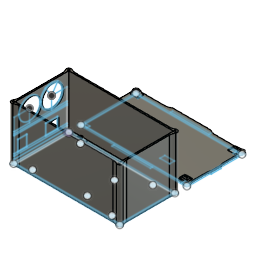
(CAD) Case Shield DMX Arduino Mega (Autodesk Fusion 360 design; units mm, degrees)
Autodesk Fusion 360 part; units mm, degrees
ref_plane "Plan de construction1" through (0, 0, 0) normal (0, 1, 0) x (0, 0, 1)
sketch "Esquisse1" plane through (0, 0, 0) normal (0, 1, 0) x (1, 0, 0)
  line L0 (0, 0) -> (108, 0)
  line L1 (108, 0) -> (108, -55)
  line L2 (108, -55) -> (0, -55)
  line L3 (0, -55) -> (0, 0)
  circle A0 centre (14, -51.75) radius 1
  circle A1 centre (15.25, -3.25) radius 1
  circle A2 centre (90.5, -3) radius 1
  circle A3 centre (96.75, -51.75) radius 1
  circle A4 centre (66, -18.5) radius 1
  circle A5 centre (66, -46.75) radius 1
  line L4 (-0.5, 0.5) -> (108.5, 0.5)
  line L5 (108.5, 0.5) -> (108.5, -55.5)
  line L6 (108.5, -55.5) -> (-0.5, -55.5)
  line L7 (-0.5, -55.5) -> (-0.5, 0.5)
  line L8 (-2, 2) -> (110, 2)
  line L9 (110, 2) -> (110, -57)
  line L10 (110, -57) -> (-2, -57)
  line L11 (-2, -57) -> (-2, 2)
  circle A6 centre (109.25, 1.25) radius 1
  circle A7 centre (109.25, 1.25) radius 2.5
  circle A8 centre (-1.25, 1.25) radius 1
  circle A9 centre (-1.25, 1.25) radius 2.5
  circle A10 centre (-1.25, -56.25) radius 1
  circle A11 centre (-1.25, -56.25) radius 2.5
  circle A12 centre (109.25, -56.25) radius 1
  circle A13 centre (109.25, -56.25) radius 2.5
  circle A14 centre (15.25, -3.25) radius 2
  circle A15 centre (66, -18.5) radius 2
  circle A16 centre (90.5, -3) radius 2
  circle A17 centre (96.75, -51.75) radius 2
  circle A18 centre (66, -46.75) radius 2
  circle A19 centre (14, -51.75) radius 2
  circle A20 centre (15.25, -3.25) radius 1.4
  circle A21 centre (90.5, -3) radius 1.4
  circle A22 centre (66, -18.5) radius 1.4
  circle A23 centre (96.75, -51.75) radius 1.4
  circle A24 centre (66, -46.75) radius 1.4
  circle A25 centre (14, -51.75) radius 1.4
  dimension "d23" = 2.8
  dimension "d24" = 2.8
  dimension "d25" = 2.8
  dimension "d26" = 2.8
  dimension "d27" = 2.8
  dimension "d28" = 2.8
  constraint horizontal L0
  constraint vertical L1
  constraint horizontal L2
  constraint vertical L3
  constraint coincident L0.start L3.end
  constraint horizontal L4
  constraint vertical L5
  constraint horizontal L6
  constraint vertical L7
  constraint horizontal L8
  constraint vertical L9
  constraint horizontal L10
  constraint vertical L11
  constraint concentric A6 A7
  constraint concentric A8 A9
  constraint concentric A10 A11
  constraint concentric A12 A13
  constraint concentric A1 A14
  constraint concentric A4 A15
  constraint concentric A2 A16
  constraint concentric A3 A17
  constraint concentric A5 A18
  constraint concentric A0 A19
  constraint concentric A1 A20
  constraint concentric A16 A21
  constraint concentric A4 A22
  constraint concentric A17 A23
  constraint concentric A18 A24
  constraint concentric A0 A25
  measures "d23" diameter of A20
  measures "d24" diameter of A21
  measures "d25" diameter of A22
  measures "d26" diameter of A23
  measures "d27" diameter of A24
  measures "d28" diameter of A25
extrude "Extrusion1" add sketch "Esquisse1" along normal blind 3 contours L0 L3 L4 L7 A9 | L0 L3 A9 | L0 L4 A7 A9 | L0 L1 L2 L3 A7 A9 A11 A13 | L3 L7 A9 A11 | L0 L1 L4 L5 A7 | L0 L1 A7 | L4 L8 A7 A9 | L4 L7 L8 L11 A8 A9 | L2 L3 A11 | L2 L3 L6 L7 A11 | L7 L11 A9 A11 | L4 L5 L8 L9 A6 A7 | L1 L5 A7 A13 | L2 L6 A11 A13 | L6 L7 L10 L11 A10 A11 | L8 L11 A8 A9 | L8 L9 A6 A7 | L1 L2 L5 L6 A13 | L1 L2 A13 | L5 L9 A7 A13 | L6 L10 A11 A13 | L10 L11 A10 A11 | L11 A8 | L8 L11 A8 | L8 A6 | L8 L9 A6 | L5 L6 L9 L10 A12 A13 | L8 A8 | L10 L11 A10 | L11 A10 | L8 L11 A8 | L8 L9 A6 | L9 A6 | L9 L10 A12 A13 | L10 L11 A10 | L10 A10 | L9 A12 | L9 L10 A12 | L10 A12 | L9 L10 A12 | A0 | A1 | A2 | A3 | A4 | A5 | A14 | A15 | A16 | A17 | A18 | A19 | A20 | A21 | A22 | A23 | A24 | A25 makes body 1
extrude "Extrusion2" add sketch "Esquisse1" along normal blind 56 contours L4 L8 A7 A9 | L4 L7 L8 L11 A8 A9 | L7 L11 A9 A11 | L4 L5 L8 L9 A6 A7 | L6 L7 L10 L11 A10 A11 | L8 L11 A8 A9 | L8 L9 A6 A7 | L5 L9 A7 A13 | L6 L10 A11 A13 | L10 L11 A10 A11 | L5 L6 L9 L10 A12 A13 | L8 L11 A8 | L8 L9 A6 | L9 L10 A12 A13 | L10 L11 A10 | L9 L10 A12 picked at (-1.9713, 1.9713) picked at (109.9713, 1.9713) picked at (-1.9713, -56.9713) picked at (109.9713, -56.9713) bodies 1
extrude "Extrusion3" add sketch "Esquisse1" along normal blind 40 contours L11 A8 | L8 L11 A8 | L8 A6 | L8 L9 A6 | L8 A8 | L10 L11 A10 | L11 A10 | L9 A6 | L10 A10 | L9 A12 | L9 L10 A12 | L10 A12 picked at (-1.4965, 1.4664) picked at (109.2357, 1.417) picked at (-1.3833, -56.1083) picked at (109.4133, -56.1968) bodies 1
extrude "Extrusion4" add sketch "Esquisse1" along normal blind 6 contours A14 | A15 | A16 | A17 | A18 | A19 | A20 | A21 | A22 | A23 | A24 | A25 bodies 1
ref_plane "Plan de construction2" through (-2, 28, 27.5) normal (-1, 0, 0) x (0, 0, 1)
sketch "Esquisse2" plane through (-2, 0, 0) normal (-1, 0, 0) x (0, 0, 1)
  line L0 (0, 0) -> (55, 0)
  line L1 (55, 0) -> (55, 3)
  line L2 (55, 3) -> (0, 3)
  line L3 (0, 3) -> (0, 0)
  line L4 (0, 3) -> (55, 3)
  line L5 (55, 3) -> (55, 6)
  line L6 (55, 6) -> (0, 6)
  line L7 (0, 6) -> (0, 3)
  line L8 (0, 6) -> (55, 6)
  line L9 (55, 6) -> (55, 8)
  line L10 (55, 8) -> (0, 8)
  line L11 (0, 8) -> (0, 6)
  line L12 (10, 8) -> (22, 8)
  line L13 (22, 8) -> (22, 19)
  line L14 (22, 19) -> (10, 19)
  line L15 (10, 19) -> (10, 8)
  line L16 (51, 8) -> (42, 8)
  line L17 (42, 8) -> (42, 19)
  line L18 (42, 19) -> (51, 19)
  line L19 (51, 19) -> (51, 8)
  line L20 (9.8, 19.2) -> (22.2, 19.2)
  line L21 (22.2, 19.2) -> (22.2, 7.8)
  line L22 (22.2, 7.8) -> (9.8, 7.8)
  line L23 (9.8, 7.8) -> (9.8, 19.2)
  line L24 (41.8, 7.8) -> (51.2, 7.8)
  line L25 (51.2, 7.8) -> (51.2, 19.2)
  line L26 (51.2, 19.2) -> (41.8, 19.2)
  line L27 (41.8, 19.2) -> (41.8, 7.8)
  line L28 (0, 8) -> (55, 8)
  line L29 (55, 8) -> (55, 24.5)
  line L30 (55, 24.5) -> (0, 24.5)
  line L31 (0, 24.5) -> (0, 8)
  line L32 (0, 24.5) -> (55, 24.5)
  line L33 (55, 24.5) -> (55, 26)
  line L34 (55, 26) -> (0, 26)
  line L35 (0, 26) -> (0, 24.5)
  line L36 (0, 26) -> (55, 26)
  line L37 (55, 26) -> (55, 28)
  line L38 (55, 28) -> (0, 28)
  line L39 (0, 28) -> (0, 26)
  line L40 (0, 28) -> (16, 28)
  line L41 (16, 28) -> (16, 41)
  line L42 (16, 41) -> (0, 41)
  line L43 (0, 41) -> (0, 28)
  line L44 (55, 28) -> (39, 28)
  line L45 (39, 28) -> (39, 41)
  line L46 (39, 41) -> (55, 41)
  line L47 (55, 41) -> (55, 28)
  circle A0 centre (16, 41) radius 11
  circle A1 centre (39, 41) radius 11
  circle A2 centre (16, 41) radius 11.1
  circle A3 centre (39, 41) radius 11.1
  circle A4 centre (16, 41) radius 12
  line L48 (9.4651, 51.0645) -> (22.5349, 51.0645)
  line L49 (16, 41) -> (22.5349, 51.0645)
  line L50 (16, 41) -> (9.4651, 51.0645)
  constraint horizontal L0
  constraint vertical L1
  constraint horizontal L2
  constraint vertical L3
  constraint coincident L0.start L3.end
  constraint horizontal L4
  constraint vertical L5
  constraint horizontal L6
  constraint vertical L7
  constraint horizontal L8
  constraint vertical L9
  constraint horizontal L10
  constraint vertical L11
  constraint horizontal L12
  constraint vertical L13
  constraint horizontal L14
  constraint vertical L15
  constraint coincident L10 L12.start
  constraint horizontal L16
  constraint vertical L17
  constraint horizontal L18
  constraint vertical L19
  constraint coincident L10 L16.start
  constraint horizontal L20
  constraint vertical L21
  constraint horizontal L22
  constraint vertical L23
  constraint horizontal L24
  constraint vertical L25
  constraint horizontal L26
  constraint vertical L27
  constraint horizontal L28
  constraint vertical L29
  constraint horizontal L30
  constraint vertical L31
  constraint horizontal L32
  constraint vertical L33
  constraint horizontal L34
  constraint vertical L35
  constraint horizontal L36
  constraint vertical L37
  constraint horizontal L38
  constraint vertical L39
  constraint horizontal L40
  constraint vertical L41
  constraint horizontal L42
  constraint vertical L43
  constraint horizontal L44
  constraint vertical L45
  constraint horizontal L46
  constraint vertical L47
  constraint coincident L41.end L42.start
  constraint coincident L45.end L46.start
  constraint concentric A0 A2
  constraint concentric A1 A3
  constraint concentric A2 A4
  constraint coincident A4 L48.start
  constraint coincident A4 L48.end
  constraint horizontal L48
extrude "Extrusion5" cut sketch "Esquisse2" against normal blind 2 contours L10 L13 L14 L15 L20 L21 L23 L28 | L10 L12 L21 L22 L23 L28 | L10 L12 L13 L14 L15 L28 bodies 1
extrude "Extrusion6" cut sketch "Esquisse2" against normal blind 2 contours L10 L16 L24 L25 L27 L28 | L10 L17 L18 L19 L25 L26 L27 L28 | L10 L16 L17 L18 L19 L28 bodies 1
extrude "Extrusion7" cut sketch "Esquisse2" against normal blind 2 contours L41 L42 A0 A2 | L41 A0 A2 L49 | L42 A0 A2 L50 | A2 A4 L48 | A2 L48 L50 | L41 L42 A0 | L41 A0 L49 | L42 A0 L50 | A0 A2 L48 L50 | A2 L48 L49 | A0 A2 L48 | A0 L48 L49 L50 | A0 A2 L48 L49 | A0 L48 bodies 1
extrude "Extrusion8" cut sketch "Esquisse2" against normal blind 2 contours L45 A1 A3 A4 | L45 L46 A1 A3 | L46 A1 A3 A4 | A3 A4 | L45 L46 A1 | L45 L46 A1 bodies 1
fillet "Congé1" radius 10 8 edges at (-2, 28, 1.1348) (-2, 28, 53.8652) (1.1348, 28, -2) (106.8651, 28, -2) (110, 28, 1.1348) (110, 28, 53.8652) (1.1348, 28, 57) (106.8652, 28, 57) on bodies 1
fillet "Congé2" radius 3 6 edges at (13.3853, 3, 2.5268) (64.1353, 3, 17.7768) (88.6353, 3, 2.2768) (94.8853, 3, 51.0268) (64.1353, 3, 46.0268) (12.1353, 3, 51.0268) on bodies 1
extrude "Extrusion9" add sketch "Esquisse1" along normal blind 7.5 contours A20 | A21 | A22 | A23 | A24 | A25 bodies 1
extrude "Extrusion10" cut 2 faces at (15.1064, 7.5, 52.36) (16.5115, 7.5, 3.3196) along direction (0, -1, 0) blind 1.5 on bodies 1 bodies 1
sketch "Esquisse3" plane through (0, 0, 0) normal (0, 1, 0) x (1, 0, 0)
  circle A0 centre (-1.25, 13.75) radius 2.5
  circle A1 centre (-1.25, 13.75) radius 1
  line L0 (110, 13) -> (-2, 13)
  line L1 (-2, 13) -> (-2, 72)
  line L2 (108.6, 14.4) -> (-0.6, 14.4)
  line L3 (-0.6, 14.4) -> (-0.6, 70.6)
  line L4 (108, 15) -> (0, 15)
  line L5 (0, 15) -> (0, 70)
  circle A2 centre (-1.25, 71.25) radius 2.5
  circle A3 centre (-1.25, 71.25) radius 1
  line L6 (-0.6, 70.6) -> (108.6, 70.6)
  line L7 (-2, 72) -> (110, 72)
  line L8 (0, 70) -> (108, 70)
  circle A4 centre (109.25, 71.25) radius 2.5
  line L9 (108, 70) -> (108, 15)
  line L10 (108.6, 70.6) -> (108.6, 14.4)
  line L11 (110, 72) -> (110, 13)
  circle A5 centre (109.25, 71.25) radius 1
  circle A6 centre (109.25, 13.75) radius 2.5
  circle A7 centre (109.25, 13.75) radius 1
  line L12 (74, 72) -> (34, 72)
  line L13 (34, 72) -> (34, 74)
  line L14 (34, 74) -> (74, 74)
  line L15 (74, 74) -> (74, 72)
  line L16 (74, 13) -> (34, 13)
  line L17 (34, 13) -> (34, 11)
  line L18 (34, 11) -> (74, 11)
  line L19 (74, 11) -> (74, 13)
  line L20 (110, 47.5) -> (111, 47.5)
  line L21 (111, 47.5) -> (111, 37.5)
  line L22 (111, 37.5) -> (110, 37.5)
  line L23 (110, 37.5) -> (110, 47.5)
  line L24 (108.6, 70.6) -> (103.6, 70.6)
  line L25 (103.6, 70.6) -> (103.6, 67.6)
  line L26 (103.6, 67.6) -> (108.6, 67.6)
  line L27 (108.6, 67.6) -> (108.6, 70.6)
  line L28 (108.6, 14.4) -> (103.5, 14.4)
  line L29 (103.5, 14.4) -> (103.5, 17.5)
  line L30 (103.5, 17.5) -> (108.6, 17.5)
  line L31 (108.6, 17.5) -> (108.6, 14.4)
  line L32 (-0.6, 14.4) -> (4.4, 14.4)
  line L33 (4.4, 14.4) -> (4.4, 17.4)
  line L34 (4.4, 17.4) -> (-0.6, 17.4)
  line L35 (-0.6, 17.4) -> (-0.6, 14.4)
  line L36 (-0.6, 70.6) -> (4.5, 70.6)
  line L37 (4.5, 70.6) -> (4.5, 67.5)
  line L38 (4.5, 67.5) -> (-0.6, 67.5)
  line L39 (-0.6, 67.5) -> (-0.6, 70.6)
  line L40 (70, 25) -> (80, 25)
  line L41 (80, 25) -> (80, 30)
  line L42 (80, 30) -> (70, 30)
  line L43 (70, 30) -> (70, 25)
  constraint horizontal L8
  constraint vertical L9
  constraint horizontal L4
  constraint vertical L5
  constraint horizontal L6
  constraint vertical L10
  constraint horizontal L2
  constraint vertical L3
  constraint horizontal L7
  constraint vertical L11
  constraint horizontal L0
  constraint vertical L1
  constraint concentric A4 A5
  constraint concentric A2 A3
  constraint concentric A0 A1
  constraint concentric A6 A7
  constraint horizontal L12
  constraint vertical L13
  constraint horizontal L14
  constraint vertical L15
  constraint coincident L7 L12.start
  constraint horizontal L16
  constraint vertical L17
  constraint horizontal L18
  constraint vertical L19
  constraint coincident L0 L16.start
  constraint horizontal L20
  constraint vertical L21
  constraint horizontal L22
  constraint vertical L23
  constraint coincident L11 L20.start
  constraint horizontal L24
  constraint vertical L25
  constraint horizontal L26
  constraint vertical L27
  constraint horizontal L28
  constraint vertical L29
  constraint horizontal L30
  constraint vertical L31
  constraint horizontal L32
  constraint vertical L33
  constraint horizontal L34
  constraint vertical L35
  constraint horizontal L36
  constraint vertical L37
  constraint horizontal L38
  constraint vertical L39
  constraint horizontal L40
  constraint vertical L41
  constraint horizontal L42
  constraint vertical L43
extrude "Extrusion12" add sketch "Esquisse3" along normal blind 3 separate body contours A0 A1 L0 L2 L32 | A0 L0 L2 A6 L16 L28 L32 | A0 A1 L2 L3 L4 L5 L32 L35 | A0 L2 L4 L32 L33 | A0 A1 L0 L1 | A0 L4 L5 | A0 L4 L5 L33 L34 | L2 L4 L29 L33 | A1 L2 L3 L32 L35 | A1 L0 L1 L2 L3 L32 L35 | A0 L1 L3 A2 L35 L39 | A0 A1 L1 L3 L35 | L0 L16 L17 L18 L19 | A1 L0 | A0 L3 L5 L34 L35 | L4 L5 L8 L9 L25 L26 L29 L30 L33 L34 L37 L38 | L2 L4 A6 L28 L29 | A1 L1 | L1 A2 A3 L7 | L1 L3 A2 A3 L39 | A1 L0 L1 | L3 L5 L34 L38 | L4 L9 A6 L29 L30 | L2 L4 L9 L10 A6 A7 L28 L31 | L0 L2 A6 A7 L28 | L1 A3 | L1 L3 A3 L6 L7 L36 L39 | A2 L6 L7 A4 L12 L24 L36 | A2 A3 L6 L7 L36 | L3 L5 A2 L38 L39 | L3 L5 A2 A3 L6 L8 L36 L39 | L0 L11 A6 A7 | L5 A2 L8 L37 L38 | L4 L9 A6 | L2 L10 A7 L28 L31 | L0 L2 L10 L11 A7 L28 L31 | L1 A3 L7 | L3 A3 L6 L36 L39 | A3 L7 | L7 L12 L13 L14 L15 | L5 A2 L8 | L0 A7 | L9 L10 A6 L30 L31 | L9 L10 L26 L30 | L10 L11 A6 A7 L31 | A2 L6 L8 L36 L37 | L0 L11 A7 | A4 L10 L11 A6 L23 L27 L31 | L6 L8 L25 L37 | L8 A4 L9 L25 L26 | A4 L9 L10 L26 L27 | L11 A7 | L7 A4 L11 A5 | L6 L7 A4 A5 L24 | L11 L20 L21 L22 L23 | L6 L8 A4 L24 L25 | L6 L8 A4 L9 L10 A5 L24 L27 | L8 A4 L9 | L7 A5 | L6 L7 L10 L11 A5 L24 L27 | A4 L10 L11 A5 L27 | L7 L11 A5 | L6 L10 A5 L24 L27 | L11 A5 | L40 L41 L42 L43 makes body 2
extrude "Extrusion14" add sketch "Esquisse3" along normal blind 6 contours A0 A1 L2 L3 L4 L5 L32 L35 | A0 L2 L4 L32 L33 | A0 L4 L5 | A0 L4 L5 L33 L34 | A1 L2 L3 L32 L35 | A0 L3 L5 L34 L35 | L2 L4 A6 L28 L29 | L4 L9 A6 L29 L30 | L2 L4 L9 L10 A6 A7 L28 L31 | L3 L5 A2 L38 L39 | L3 L5 A2 A3 L6 L8 L36 L39 | L5 A2 L8 L37 L38 | L4 L9 A6 | L2 L10 A7 L28 L31 | L3 A3 L6 L36 L39 | L5 A2 L8 | L9 L10 A6 L30 L31 | A2 L6 L8 L36 L37 | L8 A4 L9 L25 L26 | A4 L9 L10 L26 L27 | L6 L8 A4 L24 L25 | L6 L8 A4 L9 L10 A5 L24 L27 | L8 A4 L9 | L6 L10 A5 L24 L27 bodies 2
fillet "Congé5" radius 3 8 edges at (103.6, 3, -69.1) (106.1, 3, -67.6) (106.05, 3, -17.5) (103.5, 3, -15.95) (1.9, 3, -17.4) (4.4, 3, -15.9) (4.5, 3, -69.05) (1.95, 3, -67.5) on bodies 2
fillet "Congé6" radius 1 16 edges at (1.95, 6, -67.5) (4.5, 6, -69.05) (106.1, 6, -67.6) (103.6, 6, -69.1) (106.05, 6, -17.5) (103.5, 6, -15.95) (4.4, 6, -15.9) (1.9, 6, -17.4) (1.9, 6, -14.4) (-0.6, 6, -15.9) (-0.6, 6, -69.05) (1.95, 6, -70.6) (108.6, 6, -69.1) (106.1, 6, -70.6) (108.6, 6, -15.95) (106.05, 6, -14.4) on bodies 2
sketch "Esquisse5" plane through (0, 0, 0) normal (0, 1, 0) x (1, 0, 0)
  line L0 (28.2514, 49.5096) -> (17.7194, 49.5096)
  spline S0 degree 3 poles (17.7194, 49.5096) (16.7825, 49.5096) (15.9641, 49.1585) (15.2614, 48.456) knots 0 0 0 0 1 1 1 1
  spline S1 degree 3 poles (15.2614, 48.456) (14.5587, 47.754) (14.2084, 46.9338) (14.2084, 45.9959) knots 0 0 0 0 1 1 1 1
  line L1 (14.2084, 45.9959) -> (14.2084, 35.4533)
  line L2 (14.2084, 35.4533) -> (19.4601, 35.4533)
  line L3 (19.4601, 35.4533) -> (19.4601, 45.993)
  spline S2 degree 3 poles (19.4601, 45.993) (19.4601, 46.4489) (19.6379, 46.8558) (19.9956, 47.2135) knots 0 0 0 0 1 1 1 1
  spline S3 degree 3 poles (19.9956, 47.2135) (20.352, 47.5704) (20.7605, 47.749) (21.2188, 47.749) knots 0 0 0 0 1 1 1 1
  line L4 (21.2188, 47.749) -> (28.2517, 47.749)
  line L5 (28.2517, 47.749) -> (28.2514, 49.5096)
  spline S4 degree 3 poles (84.0872, 45.9969) (84.0872, 46.9346) (83.7348, 47.754) (83.0321, 48.4565) knots 0 0 0 0 1 1 1 1
  spline S5 degree 3 poles (83.0321, 48.4565) (82.3296, 49.1585) (81.5096, 49.5096) (80.5728, 49.5096) knots 0 0 0 0 1 1 1 1
  line L6 (80.5728, 49.5096) -> (70.0302, 49.5096)
  line L7 (70.0302, 49.5096) -> (70.0302, 47.7493)
  line L8 (70.0302, 47.7493) -> (77.0744, 47.7493)
  spline S6 degree 3 poles (77.0744, 47.7493) (77.5438, 47.7493) (77.9547, 47.5739) (78.3074, 47.2217) knots 0 0 0 0 1 1 1 1
  spline S7 degree 3 poles (78.3074, 47.2217) (78.659, 46.8711) (78.835, 46.4608) (78.835, 45.993) knots 0 0 0 0 1 1 1 1
  spline S8 degree 3 poles (78.835, 45.993) (78.835, 45.3479) (78.0719, 44.7463) (76.5461, 44.1832) knots 0 0 0 0 1 1 1 1
  spline S9 degree 3 poles (76.5461, 44.1832) (74.1751, 43.3053) (72.7654, 42.7368) (72.3196, 42.4796) knots 0 0 0 0 1 1 1 1
  spline S10 degree 3 poles (72.3196, 42.4796) (70.7927, 41.5898) (70.0302, 40.4185) (70.0302, 38.967) knots 0 0 0 0 1 1 1 1
  spline S11 degree 3 poles (70.0302, 38.967) (70.0302, 38.0306) (70.3813, 37.2104) (71.0843, 36.5082) knots 0 0 0 0 1 1 1 1
  spline S12 degree 3 poles (71.0843, 36.5082) (71.7865, 35.806) (72.6069, 35.4536) (73.5444, 35.4536) knots 0 0 0 0 1 1 1 1
  line L9 (73.5444, 35.4536) -> (84.0872, 35.4536)
  line L10 (84.0872, 35.4536) -> (84.0872, 37.2146)
  line L11 (84.0872, 37.2146) -> (77.0429, 37.2146)
  spline S13 degree 3 poles (77.0429, 37.2146) (76.573, 37.2146) (76.1616, 37.3914) (75.8095, 37.7422) knots 0 0 0 0 1 1 1 1
  spline S14 degree 3 poles (75.8095, 37.7422) (75.457, 38.0936) (75.2811, 38.5037) (75.2811, 38.9715) knots 0 0 0 0 1 1 1 1
  spline S15 degree 3 poles (75.2811, 38.9715) (75.2811, 39.6163) (76.0439, 40.2187) (77.5705, 40.7804) knots 0 0 0 0 1 1 1 1
  spline S16 degree 3 poles (77.5705, 40.7804) (79.9422, 41.6596) (81.3509, 42.2266) (81.7972, 42.4846) knots 0 0 0 0 1 1 1 1
  spline S17 degree 3 poles (81.7972, 42.4846) (83.3231, 43.3747) (84.0872, 44.5452) (84.0872, 45.9969) knots 0 0 0 0 1 1 1 1
  spline S18 degree 3 poles (31.8267, 57.2793) (31.8267, 56.7581) (32.2487, 56.3361) (32.7694, 56.3361) knots 0 0 0 0 1 1 1 1
  line L12 (32.7694, 56.3361) -> (36.4201, 56.3361)
  spline S19 degree 3 poles (36.4201, 56.3361) (36.9416, 56.3361) (37.3636, 56.7583) (37.3636, 57.2793) knots 0 0 0 0 1 1 1 1
  spline S20 degree 3 poles (37.3636, 57.2793) (37.3636, 57.8005) (36.9416, 58.2231) (36.4201, 58.2231) knots 0 0 0 0 1 1 1 1
  line L13 (36.4201, 58.2231) -> (32.7694, 58.2231)
  spline S21 degree 3 poles (32.7694, 58.2231) (32.2487, 58.2231) (31.8267, 57.8003) (31.8267, 57.2793) knots 0 0 0 0 1 1 1 1
  spline S22 degree 3 poles (31.8267, 54.3771) (31.8267, 53.8551) (32.2487, 53.4331) (32.7694, 53.4331) knots 0 0 0 0 1 1 1 1
  line L14 (32.7694, 53.4331) -> (36.4201, 53.4331)
  spline S23 degree 3 poles (36.4201, 53.4331) (36.9416, 53.4331) (37.3636, 53.8553) (37.3636, 54.3771) knots 0 0 0 0 1 1 1 1
  spline S24 degree 3 poles (37.3636, 54.3771) (37.3636, 54.8978) (36.9416, 55.3195) (36.4201, 55.3195) knots 0 0 0 0 1 1 1 1
  line L15 (36.4201, 55.3195) -> (32.7694, 55.3195)
  spline S25 degree 3 poles (32.7694, 55.3195) (32.2487, 55.3195) (31.8267, 54.8978) (31.8267, 54.3771) knots 0 0 0 0 1 1 1 1
  spline S26 degree 3 poles (31.8267, 51.4736) (31.8267, 50.9526) (32.2487, 50.5301) (32.7694, 50.5301) knots 0 0 0 0 1 1 1 1
  line L16 (32.7694, 50.5301) -> (36.4201, 50.5301)
  spline S27 degree 3 poles (36.4201, 50.5301) (36.9416, 50.5301) (37.3636, 50.9529) (37.3636, 51.4736) knots 0 0 0 0 1 1 1 1
  spline S28 degree 3 poles (37.3636, 51.4736) (37.3636, 51.9945) (36.9416, 52.4171) (36.4201, 52.4171) knots 0 0 0 0 1 1 1 1
  line L17 (36.4201, 52.4171) -> (32.7694, 52.4171)
  spline S29 degree 3 poles (32.7694, 52.4171) (32.2487, 52.4173) (31.8267, 51.9945) (31.8267, 51.4736) knots 0 0 0 0 1 1 1 1
  spline S30 degree 3 poles (31.8267, 48.5713) (31.8267, 48.0501) (32.2487, 47.6278) (32.7694, 47.6278) knots 0 0 0 0 1 1 1 1
  line L18 (32.7694, 47.6278) -> (36.4201, 47.6278)
  spline S31 degree 3 poles (36.4201, 47.6278) (36.9416, 47.6278) (37.3636, 48.0504) (37.3636, 48.5713) knots 0 0 0 0 1 1 1 1
  spline S32 degree 3 poles (37.3636, 48.5713) (37.3636, 49.092) (36.9416, 49.5143) (36.4201, 49.5143) knots 0 0 0 0 1 1 1 1
  line L19 (36.4201, 49.5143) -> (32.7694, 49.5143)
  spline S33 degree 3 poles (32.7694, 49.5143) (32.2487, 49.5143) (31.8267, 49.0918) (31.8267, 48.5713) knots 0 0 0 0 1 1 1 1
  line L20 (31.955, 35.4499) -> (37.2054, 35.4499)
  line L21 (37.2054, 35.4499) -> (37.2054, 45.9104)
  line L22 (37.2054, 45.9104) -> (31.955, 45.9104)
  line L23 (31.955, 45.9104) -> (31.955, 35.4499)
  spline S34 degree 3 poles (66.4683, 27.682) (66.4683, 28.2032) (66.0471, 28.6249) (65.5256, 28.6249) knots 0 0 0 0 1 1 1 1
  line L24 (65.5256, 28.6249) -> (61.8754, 28.6249)
  spline S35 degree 3 poles (61.8754, 28.6249) (61.355, 28.6249) (60.9319, 28.2029) (60.9319, 27.682) knots 0 0 0 0 1 1 1 1
  spline S36 degree 3 poles (60.9319, 27.682) (60.9319, 27.1607) (61.3553, 26.7385) (61.8754, 26.7385) knots 0 0 0 0 1 1 1 1
  line L25 (61.8754, 26.7385) -> (65.5256, 26.7385)
  spline S37 degree 3 poles (65.5256, 26.7385) (66.0471, 26.7385) (66.4683, 27.1607) (66.4683, 27.682) knots 0 0 0 0 1 1 1 1
  spline S38 degree 3 poles (66.4683, 30.5844) (66.4683, 31.1059) (66.0471, 31.5279) (65.5256, 31.5279) knots 0 0 0 0 1 1 1 1
  line L26 (65.5256, 31.5279) -> (61.8754, 31.5279)
  spline S39 degree 3 poles (61.8754, 31.5279) (61.355, 31.5279) (60.9319, 31.1059) (60.9319, 30.5844) knots 0 0 0 0 1 1 1 1
  spline S40 degree 3 poles (60.9319, 30.5844) (60.9319, 30.0637) (61.3553, 29.6417) (61.8754, 29.6417) knots 0 0 0 0 1 1 1 1
  line L27 (61.8754, 29.6417) -> (65.5256, 29.6417)
  spline S41 degree 3 poles (65.5256, 29.6417) (66.0471, 29.6417) (66.4683, 30.0637) (66.4683, 30.5844) knots 0 0 0 0 1 1 1 1
  spline S42 degree 3 poles (66.4683, 33.4877) (66.4683, 34.0084) (66.0471, 34.4307) (65.5256, 34.4307) knots 0 0 0 0 1 1 1 1
  line L28 (65.5256, 34.4307) -> (61.8754, 34.4307)
  spline S43 degree 3 poles (61.8754, 34.4307) (61.355, 34.4307) (60.9319, 34.0084) (60.9319, 33.4877) knots 0 0 0 0 1 1 1 1
  spline S44 degree 3 poles (60.9319, 33.4877) (60.9319, 32.9665) (61.3553, 32.5442) (61.8754, 32.5442) knots 0 0 0 0 1 1 1 1
  line L29 (61.8754, 32.5442) -> (65.5256, 32.5442)
  spline S45 degree 3 poles (65.5256, 32.5442) (66.0471, 32.5442) (66.4683, 32.9665) (66.4683, 33.4877) knots 0 0 0 0 1 1 1 1
  spline S46 degree 3 poles (66.4683, 36.3902) (66.4683, 36.9112) (66.0471, 37.3337) (65.5256, 37.3337) knots 0 0 0 0 1 1 1 1
  line L30 (65.5256, 37.3337) -> (61.8754, 37.3337)
  spline S47 degree 3 poles (61.8754, 37.3337) (61.355, 37.3337) (60.9319, 36.9112) (60.9319, 36.3902) knots 0 0 0 0 1 1 1 1
  spline S48 degree 3 poles (60.9319, 36.3902) (60.9319, 35.869) (61.3553, 35.4467) (61.8754, 35.4467) knots 0 0 0 0 1 1 1 1
  line L31 (61.8754, 35.4467) -> (65.5256, 35.4467)
  spline S49 degree 3 poles (65.5256, 35.4467) (66.0471, 35.447) (66.4683, 35.8692) (66.4683, 36.3902) knots 0 0 0 0 1 1 1 1
  line L32 (66.3411, 49.5111) -> (61.0894, 49.5111)
  line L33 (61.0894, 49.5111) -> (61.0894, 39.0514)
  line L34 (61.0894, 39.0514) -> (66.3411, 39.0514)
  line L35 (66.3411, 39.0514) -> (66.3411, 49.5111)
  line L36 (56.9508, 48.0946) -> (54.7931, 44.9645)
  spline S50 degree 3 poles (54.7931, 44.9645) (54.3605, 44.2703) (54.0697, 43.5255) (54.8299, 43.1109) knots 0 0 0 0 1 1 1 1
  spline S51 degree 3 poles (54.8299, 43.1109) (56.6827, 42.3867) (57.922, 41.0852) (57.922, 39.5964) knots 0 0 0 0 1 1 1 1
  spline S52 degree 3 poles (57.922, 39.5964) (57.922, 37.3221) (55.0352, 35.4483) (51.4755, 35.4483) knots 0 0 0 0 1 1 1 1
  line L37 (51.4755, 35.4483) -> (40.7035, 35.4483)
  line L38 (40.7035, 35.4483) -> (40.7035, 49.5059)
  line L39 (40.7035, 49.5059) -> (45.9536, 49.5059)
  line L40 (45.9536, 49.5059) -> (45.9536, 37.3382)
  line L41 (45.9536, 37.3382) -> (45.9571, 37.339)
  spline S53 degree 2 poles (45.9571, 37.339) (48.4238, 37.339) (49.5271, 37.339) knots 0 0 0 1 1 1
  spline S54 degree 3 poles (49.5271, 37.339) (51.5805, 37.339) (53.2468, 38.4029) (53.2468, 39.7152) knots 0 0 0 0 1 1 1 1
  spline S55 degree 3 poles (53.2468, 39.7152) (53.2468, 40.0623) (53.1265, 40.3915) (52.9185, 40.6883) knots 0 0 0 0 1 1 1 1
  spline S56 degree 3 poles (52.9185, 40.6883) (52.7386, 40.9707) (52.4131, 41.2837) (52.1605, 41.5226) knots 0 0 0 0 1 1 1 1
  spline S57 degree 3 poles (52.1605, 41.5226) (51.4371, 42.2084) (49.9131, 42.665) (49.4953, 42.8939) knots 0 0 0 0 1 1 1 1
  spline S58 degree 3 poles (49.4953, 42.8939) (48.7077, 43.3228) (49.0093, 44.0943) (49.4567, 44.8135) knots 0 0 0 0 1 1 1 1
  line L42 (49.4567, 44.8135) -> (52.7137, 49.5066)
  line L43 (52.7137, 49.5066) -> (57.9649, 49.5066)
  line L44 (57.9649, 49.5066) -> (56.9508, 48.0946)
extrude "Extrusion16" cut sketch "Esquisse5" along normal blind 0.5 bodies 2
extrude "Extrusion17" cut sketch "Esquisse3" along normal blind 20 contours L40 L41 L42 L43 bodies 2
fillet "Congé9" radius 10 14 edges at (-2, 1.5, -16.1348) (-2, 1.5, -68.8652) (1.1348, 1.5, -72) (106.8651, 1.5, -72) (110, 1.5, -68.8652) (110, 1.5, -16.1348) (106.8652, 1.5, -13) (1.1348, 1.5, -13) (74, 1.5, -13) (34, 1.5, -13) (34, 1.5, -72) (74, 1.5, -72) (110, 1.5, -47.5) (110, 1.5, -37.5) on bodies 2
fillet "Congé10" radius 1.5 28 edges at (110.2532, 0, -35.3772) (110, 0, -26.6349) (110.3563, 0, -17.4829) (111.0178, 0, -11.9822) (105.5171, 0, -12.6437) (91.4357, 0, -13) (76.8377, 0, -12.4868) (54, 0, -11) (31.1623, 0, -12.4868) (16.5643, 0, -13) (2.4829, 0, -12.6437) (-3.0178, 0, -11.9822) (-2.3563, 0, -17.4829) (-2, 0, -42.5) (-2.3563, 0, -67.5171) (-3.0178, 0, -73.0178) (2.4829, 0, -72.3563) (16.5643, 0, -72) (31.1623, 0, -72.5132) (54, 0, -74) (76.8377, 0, -72.5132) (91.4357, 0, -72) (105.5171, 0, -72.3563) (111.0178, 0, -73.0178) (110.3563, 0, -67.5171) (110, 0, -58.3651) (110.2532, 0, -49.6228) (111, 0, -42.5) on bodies 2
